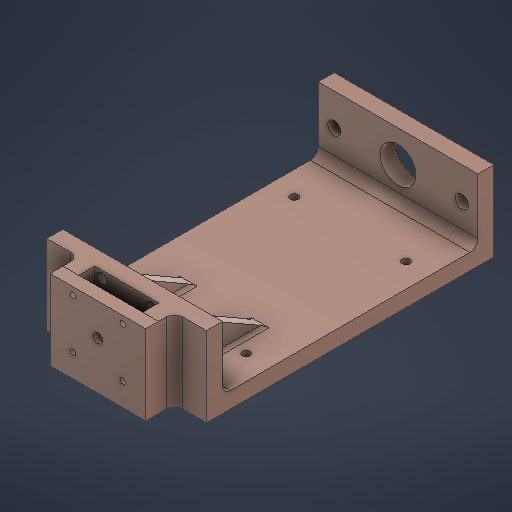
# Autodesk Inventor part: Base
Saved by Autodesk Inventor 2026 (Build 300175000, 175)
## iProperties
Created: 2025-08-18
Part Number: Base
Material: Plástico PC/ABS
Document SubType Name: Modeling
Designer: Thomas
Density: 1.1 g/cm^3
Appearance: Suave - Blanco
Author: Thomas
Autodesk Inventor part; units mm, degrees
ref_plane "YZ Plane" through (0, 0, 0) normal (1, 0, 0) x (0, 1, 0)
ref_plane "XZ Plane" through (0, 0, 0) normal (0, 1, 0) x (-1, 0, 0)
ref_plane "XY Plane" through (0, 0, 0) normal (0, 0, 1) x (1, 0, 0)
sketch "Boceto1" plane through (0, 0, 0) normal (0, 0, 1) x (1, 0, 0)
  line L0 (50, -20) -> (-50, -20)
  line L1 (-50, -20) -> (-50, 20)
  line L2 (-50, 20) -> (50, 20)
  line L3 (50, 20) -> (50, -20)
  line L4 (50, -20) -> (-50, 20) construction
  line L5 (-50, -20) -> (50, 20) construction
  circle A0 centre (40, 0) radius 4.1
  circle A1 centre (-40, 0) radius 4.1
  circle A2 centre (0, 0) radius 10
  dimension "d0" = 8.2
  dimension "d1" = 8.2
  dimension "d2" = 80
  dimension "d3" = 40
  dimension "d4" = 20
  dimension "d5" = 40
  dimension "d6" = 100
  constraints: 12 end point, 3 centre point, 2 horizontal alignment, 2 midpoint, 2 parallel, 1 coincident, 1 horizontal, 1 perpendicular
  measures "d0" diameter of A0
  measures "d1" diameter of A1
  measures "d2" distance of A1.centre A0.centre
  measures "d3" distance of point (0, 0) A0.centre
  measures "d4" diameter of A2
  measures "d5" distance of L2.end L0.start
  measures "d6" distance of L1.end L2.end
extrude "Extrusión1" add sketch "Boceto1" along normal blind 10
sketch "Boceto2" plane through (0, 0, 10) normal (0, 0, 1) x (1, 0, 0)
  circle A0 centre (-40, 0) radius 4.1 projected
  circle A1 centre (40, 0) radius 4.1 projected
  point P0 (0, 0)
extrude "Extrusión2" add sketch "Boceto2" against normal blind 2
sketch "Boceto3" plane through (0, 0, 0) normal (1, 0, 0) x (0, 1, 0)
  line L0 (20, 0) -> (-20, 0) projected
  line L1 (-20, 0) -> (-20, -160)
  line L2 (-20, -160) -> (20, -160)
  line L3 (20, -160) -> (20, -170)
  line L4 (20, -170) -> (-30, -170)
  line L5 (-30, -170) -> (-30, 10)
  line L6 (-30, 10) -> (-20, 10)
  line L7 (-20, 10) -> (20, 10) projected
  line L8 (4.1, 8) -> (-4.1, 8) projected
  line L9 (0, -170) -> (0, 30) construction
  line L10 (-20, 0) -> (-20, 10) projected
  line L11 (-20, 10) -> (-20, 0)
  point P0 (0, 0)
  dimension "d11" = 160
  dimension "d12" = 10
  dimension "d13" = 10
  dimension "d15" = 200
  dimension "d16" = 10
  constraints: 16 end point, 6 perpendicular, 2 point on line, 1 collinear, 1 vertical, 1 vertical alignment
  measures "d11" distance between parallel lines of L2 L0
  measures "d12" distance between parallel lines of L7 L0
  measures "d13" distance between parallel lines of L2 L4
  measures "d15" distance of L9.start L9.end
  measures "d16" distance between parallel lines of L1 L5
extrude "Extrusión3" add sketch "Boceto3" along normal mid plane 100
sketch "Boceto4" plane through (50, 20, -170) normal (0, 0, -1) x (-1, 0, 0)
  circle A0 centre (50, -20) radius 10 projected
  circle A1 centre (50, -20) radius 11.15
  circle A2 centre (10, -20) radius 4.1 projected
  circle A3 centre (90, -20) radius 4.1 projected
  dimension "d19" = 22.3
  constraints: 1 centre point, 1 coincident
  measures "d19" diameter of A1
extrude "Extrusión4" cut sketch "Boceto4" against normal up to surface (10 mm away) contours A0 | A1 | A2 | A3
sketch "Boceto5" plane through (0, 0, 0) normal (1, 0, 0) x (0, 1, 0)
  line L0 (-30, -170) -> (-30, 10) projected
  line L1 (-30, 10) -> (-30, 28)
  line L2 (-30, 28) -> (20.0145, 28)
  line L3 (20.0145, 28) -> (20.0145, 20)
  line L4 (20.0145, 20) -> (-20, 20)
  line L5 (-20, 20) -> (-20, 10)
  line L6 (20, 10) -> (-30, 10) projected
  point P0 (0, 0)
  point P1 (-20, 0)
  dimension "d22" = 10
  dimension "d23" = 8
  constraints: 10 end point, 4 perpendicular, 1 vertical, 1 vertical alignment
  measures "d22" distance between parallel lines of L6 L4
  measures "d23" distance of L2.end L3.end
extrude "Extrusión5" add sketch "Boceto5" along normal mid plane 60
sketch "Boceto6" plane through (-30, -30, 28) normal (0, 0, 1) x (1, 0, 0)
  circle A0 centre (30, 30) radius 10 construction
  circle A1 centre (30, 30) radius 21.9203 construction
  circle A2 centre (14.5, 45.5) radius 2.5
  line L0 (30, 30) -> (14.5, 45.5) construction
  line L1 (30, 30) -> (30, 51.9203) construction
  circle A3 centre (14.5, 14.5) radius 2.5
  circle A4 centre (45.5, 14.5) radius 2.5
  circle A5 centre (45.5, 45.5) radius 2.5
  circle A6 centre (14.5, 45.5) radius 1.75
  circle A7 centre (14.5, 14.5) radius 1.75
  circle A8 centre (45.5, 14.5) radius 1.75
  circle A9 centre (45.5, 45.5) radius 1.75
  circle A10 centre (30, 30) radius 3
  dimension "d27" = 5
  dimension "d29" = 45
  dimension "d32" = 360
  dimension "d34" = 3.5
  dimension "d37" = 360
  dimension "d49" = 31
  dimension "d60" = 6
  constraints: 10 centre point, 4 end point, 3 coincident, 2 point on circle, 1 vertical, 18 other
  measures "d27" diameter of A2
  measures "d29" angle of L1 L0
  measures "d34" diameter of A6
  measures "d49" distance of A4.centre A5.centre
  measures "d60" diameter of A10
extrude "Extrusión6" cut sketch "Boceto6" against normal up to surface (8 mm away) contours A6 | A7 | A8 | A9 | A10
sketch "Boceto7" plane through (0, 0, 0) normal (0, 0, -1) x (-1, 0, 0)
  circle A0 centre (-15.5, 15.5) radius 1.75 construction
  circle A1 centre (-15.5, 15.5) radius 3.25
  circle A2 centre (-15.5, -15.5) radius 3.25
  circle A3 centre (15.5, -15.5) radius 3.25
  circle A4 centre (15.5, 15.5) radius 3.25
  point P0 (0, 0)
  dimension "d41" = 6.5
  dimension "d44" = 360
  constraints: 4 centre point, 1 coincident, 9 other
  measures "d41" diameter of A1
extrude "Extrusión7" cut sketch "Boceto7" against normal up to surface (10 mm away)
fillet "Empalme1" radius 5 2 edges at (30, -25, 10) (-30, -25, 10)
fillet "Empalme2" radius 2 3 edges at (32.5, -20, 10) (0, -20, 10) (-32.5, -20, 10)
fillet "Empalme3" radius 5 2 edges at (0, -20, -160) (0, -20, 0)
sketch "Boceto8" plane through (-50, -20, -5) normal (0, 1, 0) x (1, 0, 0)
  circle A0 centre (85, 25) radius 2.5
  circle A1 centre (15, 25) radius 2.5
  line L0 (100, 150) -> (100, 0) projected
  line L1 (100, 75) -> (-31.9752, 75) construction
  line L2 (100, -5) -> (0, -5) projected
  circle A2 centre (85, 125) radius 2.5
  circle A3 centre (15, 125) radius 2.5
  point P0 (50, -5)
  point P1 (50, -5)
  dimension "d53" = 5
  dimension "d54" = 5
  dimension "d55" = 70
  dimension "d56" = 35
  dimension "d57" = 50
  constraints: 4 centre point, 2 end point, 2 midpoint, 2 symmetric about line, 1 horizontal, 1 horizontal alignment, 2 other
  measures "d53" diameter of A0
  measures "d54" diameter of A1
  measures "d55" distance of A1.centre A0.centre
  measures "d56" horizontal distance of point (50, -5) A1.centre
  measures "d57" distance from line of A0.centre L1
extrude "Extrusión8" cut sketch "Boceto8" against normal through all
ref_plane "Plano de trabajo1" through (26, 20, 10) normal (1, 0, 0) x (0, 0, -1)
sketch "Boceto9" plane through (26, 20, 10) normal (1, 0, 0) x (0, 0, -1)
  line L0 (10, 0) -> (10, -35) projected
  line L1 (10, -10.5) -> (61.0955, -40)
  line L2 (165, -40) -> (15, -40) projected
  arc A0 (10, -35) -> (15, -40) centre (15, -35) ccw projected
  point P0 (10, -20)
  dimension "d62" = 29.5
  dimension "d63" = 30
  constraints: 2 end point, 2 point on line
  measures "d62" distance from line of L2 L1.start
  measures "d63" angle of L1 L2
extrude "Extrusión9" add sketch "Boceto9" against normal blind 7
mirror "Simetría1" about plane through (0, 0, 0) normal (1, 0, 0) of "Extrusión9"
fillet "Empalme4" radius 2 12 edges at (26, -18.5355, -1.4645) (26, -2.75, 0) (26, -20, -28.0477) (19, -20, -28.0477) (19, -2.75, 0) (19, -18.5355, -1.4645) (-19, -18.5355, -1.4645) (-19, -2.75, 0) (-19, -20, -28.0477) (-26, -18.5355, -1.4645) (-26, -2.75, 0) (-26, -20, -28.0477)
sketch "Boceto10" plane through (-30, -20, 20) normal (0, 1, 0) x (1, 0, 0)
  line L0 (0, 0) -> (0, 5) projected
  arc A0 (0, 5) -> (-1, 8) centre (-5, 5) ccw projected
  spline S0 degree 2 poles (-5, 10) (-2.5, 10) (-1, 8) knots 0 0 0 1 1 1 weights 1 0.894427 1 projected
  line L1 (80, 10) -> (-20, 10) projected
  spline S1 degree 2 poles (61, 8) (62.5, 10) (65, 10) knots 0 0 0 1 1 1 weights 1 0.894427 1 projected
  arc A1 (61, 8) -> (60, 5) centre (65, 5) ccw projected
  line L2 (60, 5) -> (60, 0) projected
  line L3 (10, 0) -> (10, 10)
  line L4 (50, -0.1) -> (50, 10)
  line L5 (50, -0.1) -> (60, -0.1)
  line L6 (60, -8) -> (60, 5) projected
  line L7 (60, 0) -> (60, -0.1)
  line L8 (10, 0) -> (10, -0.1)
  line L9 (10, -0.1) -> (0, -0.1)
  line L10 (0, -8) -> (0, 0) projected
  line L11 (0, 0) -> (0, -0.1)
  point P0 (30, 20)
  dimension "d68" = 10
  dimension "d69" = 10
  dimension "d72" = 10.1
  dimension "d73" = 10.1
  constraints: 14 end point, 4 point on line, 3 perpendicular, 2 collinear, 1 horizontal, 1 vertical, 2 other
  measures "d68" distance between parallel lines of L0 L3
  measures "d69" distance between parallel lines of L4 L2
  measures "d72" distance of L4.start L4.end
  measures "d73" distance between parallel lines of L1 L9
extrude "Extrusión10" add sketch "Boceto10" along normal up to surface (40 mm away)
chamfer "Chaflán1" distance 1 angle 45 2 edges at (44.1, 0, -170) (-35.9, 0, -170)
sketch "Boceto12" plane through (-14.5732, -11.7381, -170) normal (-1, 0, 0) x (0, 0, 1)
  line L0 (1.5, 26.5563) -> (14.2542, 26.5563)
  line L1 (14.2542, 26.5563) -> (14.2542, -2.4606)
  line L2 (14.2542, -2.4606) -> (1.5, -2.4606)
  line L3 (1.5, -2.4606) -> (1.5, 26.5563)
  line L4 (0, 0) -> (0, 24.153) projected
  point P0 (170, 11.7381)
  dimension "d78" = 1.5
  constraints: 8 end point, 2 parallel, 1 horizontal, 1 perpendicular
  measures "d78" distance between parallel lines of L4 L3
equation "\"d1\" = d0"
equation "\"d3\" = 0.5 * d2"
equation "\"d16\" = d13"
equation "\"d54\" = d53"
equation "\"d56\" = 0.5 * d55"
equation "\"d73\" = d72"
